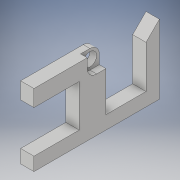
# Autodesk Inventor part: Main
Saved by Autodesk Inventor 2019 (Build 230136000, 136)
## iProperties
Created: 2018-08-02
Part Number: Main
Material: Generic
Document SubType Name: Modeling
Designer: zacha
Density: 1 g/cm^3
Appearance: Default
Author: zacha
Autodesk Inventor part; units mm, degrees
ref_plane "YZ Plane" through (0, 0, 0) normal (1, 0, 0) x (0, 1, 0)
ref_plane "XZ Plane" through (0, 0, 0) normal (0, 1, 0) x (-1, 0, 0)
ref_plane "XY Plane" through (0, 0, 0) normal (0, 0, 1) x (1, 0, 0)
sketch "Sketch1" plane through (0, 0, 0) normal (1, 0, 0) x (0, 1, 0)
  line L0 (0, 0) -> (20, 0) construction
  line L1 (20, 0) -> (20, -21.5)
  line L2 (20, -21.5) -> (0, -21.5)
  line L3 (0, -21.5) -> (0, 0)
  line L4 (20, 0) -> (27.85, 0)
  line L5 (27.85, 0) -> (27.85, -29.755)
  line L6 (27.85, -34.2) -> (26.58, -34.2) construction
  line L7 (-6.35, -34.2) -> (-6.35, 0)
  line L8 (-6.35, 0) -> (0, 0)
  line L9 (-6.35, -34.2) -> (-6.35, -59.6)
  line L10 (-6.35, -59.6) -> (20.23, -59.6)
  line L11 (20.23, -59.6) -> (20.23, -53.25) construction
  line L12 (20.23, -53.25) -> (0, -53.25)
  line L13 (0, -53.25) -> (0, -34.2)
  line L14 (0, -34.2) -> (-6.35, -34.2) construction
  line L15 (20.23, -53.25) -> (26.58, -59.6)
  line L16 (26.58, -59.6) -> (20.23, -59.6)
  line L17 (20.23, -53.25) -> (20.23, -34.2) construction
  line L18 (26.58, -59.6) -> (26.58, -34.2) construction
  circle A0 centre (23.405, -29.755) radius 3.175
  line L19 (23.405, -29.755) -> (23.405, -59.6) construction
  arc A1 (27.85, -29.755) -> (23.405, -34.2) centre (23.405, -29.755) ccw construction
  arc A2 (23.405, -34.2) -> (27.85, -29.755) centre (23.405, -29.755) ccw
  line L20 (27.85, -29.755) -> (27.85, -34.2) construction
  line L21 (26.58, -34.2) -> (23.405, -34.2) construction
  line L22 (23.405, -34.2) -> (0, -34.2)
  dimension "d0" = 20
  dimension "d1" = 21.5
  dimension "d2" = 7.85
  dimension "d3" = 12.7
  dimension "d4" = 6.35
  dimension "d5" = 25.4
  dimension "d6" = 26.58
  dimension "d7" = 6.35
  dimension "d8" = 20.23
  dimension "d11" = 6.35
  dimension "d12" = 45
  dimension "d15" = 6.35
  dimension "d16" = 3.175
  dimension "d17" = 3.175
  dimension "d19" = 8.89
  dimension "d22" = 34.2
  constraints: 46 end point, 14 perpendicular, 7 horizontal, 5 tangent, 4 point on circle, 4 point on line, 4 vertical, 3 centre point, 2 parallel, 1 coincident, 1 midpoint
  measures "d0" distance of L1.end L2.end
  measures "d1" distance of L0.end L1.end
  measures "d2" distance of L0.end L4.end
  measures "d3" distance between parallel lines of L6 L2
  measures "d4" distance between parallel lines of L7 L3
  measures "d5" distance of L7.start L9.end
  measures "d6" distance of L9.end L10.end
  measures "d7" distance of L10.end L11.end
  measures "d8" distance of L11.end L12.end
  measures "d11" distance between parallel lines of L9 L13
  measures "d12" angle of L15 L11
  measures "d15" diameter of A0
  measures "d16" distance from line of L19 L15.end
  measures "d17" distance from line of L19 L10.end
  measures "d19" diameter of A1
  measures "d22" distance between parallel lines of L7 L5
extrude "Extrusion1" add sketch "Sketch1" along normal blind 6.35
sketch "Sketch2" plane through (6.35, 0, 0) normal (1, 0, 0) x (0, 0, -1)
  arc A0 (34.2, 23.405) -> (29.755, 27.85) centre (29.755, 23.405) ccw
  arc A1 (34.2, 23.405) -> (29.755, 27.85) centre (29.755, 23.405) ccw projected
  line L0 (29.755, 18.96) -> (34.2, 18.96)
  line L1 (34.2, 0) -> (34.2, 23.405) projected
  line L2 (34.2, 18.96) -> (34.2, 23.405)
  arc A2 (29.755, 18.96) -> (34.2, 23.405) centre (29.755, 23.405) ccw construction
  line L3 (25.31, 23.405) -> (25.31, 27.85)
  line L4 (29.755, 27.85) -> (0, 27.85) projected
  line L5 (25.31, 27.85) -> (29.755, 27.85)
  arc A3 (25.31, 23.405) -> (29.755, 18.96) centre (29.755, 23.405) ccw
  arc A4 (29.755, 27.85) -> (25.31, 23.405) centre (29.755, 23.405) ccw construction
  point P0 (0, 0)
  constraints: 12 tangent, 9 end point, 8 point on circle, 4 centre point, 1 collinear, 1 concentric, 1 horizontal, 1 perpendicular, 1 point on line, 1 vertical
extrude "Extrusion2" cut sketch "Sketch2" against normal blind 3.175
equation "\"d16\" = d17"
body "Solid1"
